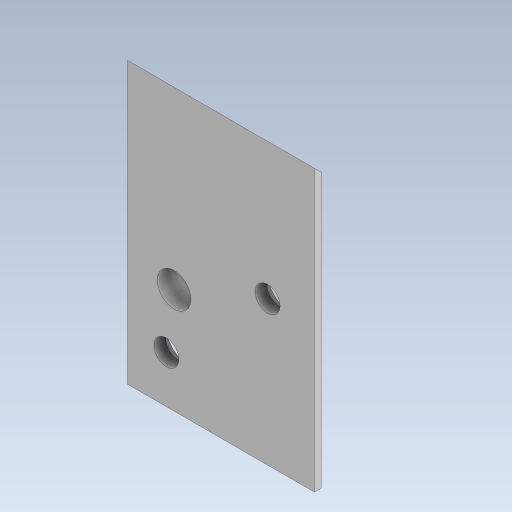
# Autodesk Inventor part: MK3_Adapter
Saved by Autodesk Inventor 2023.4 (Build 274418000, 418)
## iProperties
Created: 2024-09-25
Part Number: MK3_Adapter
Material: Generic
Document SubType Name: Modeling
Designer: dverd
Density: 1 g/cm^3
Appearance: Default
Author: dverd
Autodesk Inventor part; units mm, degrees
ref_plane "YZ Plane" through (0, 0, 0) normal (1, 0, 0) x (0, 1, 0)
ref_plane "XZ Plane" through (0, 0, 0) normal (0, 1, 0) x (-1, 0, 0)
ref_plane "XY Plane" through (0, 0, 0) normal (0, 0, 1) x (1, 0, 0)
sketch "Sketch1" plane through (0, 0, 0) normal (0, 0, 1) x (1, 0, 0)
  line L0 (0, 0) -> (24, 0)
  line L1 (24, 0) -> (24, 36)
  line L2 (24, 36) -> (0, 36)
  line L3 (0, 36) -> (0, 0)
  dimension "d0" = 24
  dimension "d1" = 36
  constraints: 8 end point, 2 parallel, 1 horizontal, 1 perpendicular
  measures "d0" distance of L2.end L1.end
  measures "d1" distance of L1.end L0.end
extrude "Extrusion1" add sketch "Sketch1" along normal blind 3
chamfer "Chamfer1" distance 2.142 angle 45 2 edges at (12, 0, 0) (24, 18, 0)
chamfer "Chamfer2" distance 3 angle 45 1 edges at (10.929, 36, 0)
sketch "Sketch4" plane through (0, 0, 0) normal (0, 0, -1) x (-1, 0, 0)
  line L0 (0, 33) -> (0, 2.142) projected
  line L1 (-24, 0) -> (0, 0) projected
  circle A0 centre (-6, 13.5) radius 6
  line L2 (0, 36) -> (0, 0) projected
  dimension "d25" = 6
  dimension "d28" = 13.5
  constraints: 1 centre point, 1 coincident, 1 tangent
  measures "d25" distance from line of L0 point (-6, 13.5)
  measures "d28" distance from line of L1 point (-6, 13.5)
extrude "Extrusion4" add sketch "Sketch4" along normal blind 6
sketch "Sketch5" plane through (6, 13.5, -6) normal (0, 0, -1) x (-1, 0, 0)
  point P0 (6, -13.5)
sketch "Sketch6" plane through (6, 13.5, -6) normal (0, 0, -1) x (-1, 0, 0)
  circle A0 centre (0, 0) radius 6 projected
  point P0 (6, -13.5)
  point P1 (6, 0)
  constraints: 1 coincident, 1 horizontal alignment
hole "Hole1" at (6, 13.5, -6) direction (0, 0, 1) diameter 4.3 end through all counterbore diameter 8.2 counterbore depth 6
sketch "Sketch7" plane through (6, 13.5, -6) normal (0, 0, -1) x (-1, 0, 0)
  line L0 (6, 0) -> (6, -11.358) projected
  line L1 (-18, -13.5) -> (6, -13.5) projected
  circle A0 centre (0, 7) radius 5
  line L2 (6, 19.5) -> (6, 0) projected
  line L3 (5, 7) -> (5, 3.3166)
  circle A1 centre (0, 0) radius 6 projected
  line L4 (-5, 7) -> (-5, 3.3166)
  point P0 (1, -7.45)
  point P1 (-12, 5)
  dimension "d46" = 5
  dimension "d47" = 6.05
  dimension "d48" = 18.5
  dimension "d49" = 18
  dimension "d57" = 10
  dimension "d58" = 20.5
  dimension "d59" = 6
  constraints: 4 end point, 4 point on circle, 1 centre point, 1 parallel, 1 tangent, 1 vertical
  measures "d46" distance from line of L0 point (1, -7.45)
  measures "d47" distance from line of L1 point (1, -7.45)
  measures "d48" distance from line of L1 point (-12, 5)
  measures "d49" distance from line of L0 point (-12, 5)
  measures "d57" diameter of A0
  measures "d58" distance from line of L1 A0.centre
  measures "d59" distance from line of L2 A0.centre
hole "Hole3" at (5, 6.05, -6) at (18, 18.5, -6) direction (0, 0, 1) diameter 3.202 end through all counterbore diameter 6.197 counterbore depth 7.5
extrude "Extrusion5" add sketch "Sketch7" against normal blind 6 contours A0 A1 | L3 A1 A0 | A0 A1 L4 picked at (0.2009, 7.9633)
body "Solid1"
